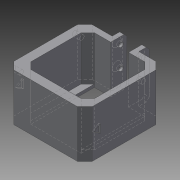
# Autodesk Inventor part: z-stepper holder
Saved by Autodesk Inventor 2015 (Build 190159000, 159)
## iProperties
Created: 2019-01-12
Part Number: z-stepper holder
Material: Generic
Document SubType Name: Modeling
Designer: Toby
Density: 1 g/cm^3
Appearance: Default
Author: Toby
Autodesk Inventor part; units mm, degrees
ref_plane "YZ Plane" through (0, 0, 0) normal (1, 0, 0) x (0, 1, 0)
ref_plane "XZ Plane" through (0, 0, 0) normal (0, 1, 0) x (-1, 0, 0)
ref_plane "XY Plane" through (0, 0, 0) normal (0, 0, 1) x (1, 0, 0)
sketch "Sketch1" plane through (0, 0, 0) normal (0, 0, 1) x (1, 0, 0)
  line L0 (-30.0725, 29.5446) -> (12.9275, 29.5446)
  line L1 (12.9275, 29.5446) -> (12.9275, -13.4554)
  line L2 (12.9275, -13.4554) -> (-30.0725, -13.4554)
  line L3 (-30.0725, -13.4554) -> (-30.0725, 29.5446)
  line L4 (-36.0725, 33.5446) -> (16.9275, 33.5446)
  line L5 (16.9275, 33.5446) -> (16.9275, -19.4554)
  line L6 (16.9275, -19.4554) -> (-36.0725, -19.4554)
  line L7 (-36.0725, -19.4554) -> (-36.0725, 33.5446)
  point P0 (0, 0)
  dimension "d0" = 43
  dimension "d1" = 43
  dimension "d2" = 6
  dimension "d3" = 4
  dimension "d4" = 6
  dimension "d5" = 4
  constraints: 16 end point, 4 parallel, 2 horizontal, 2 perpendicular
  measures "d0" distance of L2.end L0.start
  measures "d1" distance of L0.start L0.end
  measures "d2" distance between parallel lines of L7 L3
  measures "d3" distance between parallel lines of L5 L1
  measures "d4" distance between parallel lines of L6 L2
  measures "d5" distance between parallel lines of L4 L0
extrude "Extrusion1" add sketch "Sketch1" along normal blind 30
sketch "Sketch2" plane through (-36.0725, -19.4554, 0) normal (-1, 0, 0) x (0, 0, 1)
  line L0 (0, 0) -> (30, 0) projected
  point P0 (0, 19.4554)
  point P1 (25.9467, 5)
  point P2 (25.9467, 46)
  dimension "d8" = 5
  dimension "d9" = 41
  measures "d8" distance from line of L0 point (25.947, 5)
  measures "d9" distance of point (25.947, 5) point (25.947, 46)
hole "Hole1" at (-36.0725, -14.4554, 25.9467) at (-36.0725, 26.5446, 25.9467) direction (1, 0, 0) diameter 3 depth 5 tip angle 118
chamfer "Chamfer1" distance 4.5 angle 45 4 edges at (-30.0725, 29.5446, 15) (-30.0725, -13.4554, 15) (12.9275, -13.4554, 15) (12.9275, 29.5446, 15)
chamfer "Chamfer2" distance 5 angle 45 4 edges at (-36.0725, 33.5446, 15) (-36.0725, -19.4554, 15) (16.9275, -19.4554, 15) (16.9275, 33.5446, 15)
sketch "Sketch3" plane through (0, 0, 0) normal (0, 0, -1) x (-1, 0, 0)
  line L0 (-16.9275, 33.5446) -> (36.0725, 33.5446)
  line L1 (36.0725, 33.5446) -> (36.0725, -19.4554)
  line L2 (36.0725, -19.4554) -> (-16.9275, -19.4554)
  line L3 (-16.9275, -19.4554) -> (-16.9275, 33.5446)
  line L4 (31.0725, 33.5446) -> (-11.9275, 33.5446) projected
  line L5 (36.0725, -14.4554) -> (36.0725, 28.5446) projected
  line L6 (-11.9275, -19.4554) -> (31.0725, -19.4554) projected
  line L7 (-16.9275, 28.5446) -> (-16.9275, -14.4554) projected
  line L8 (-8.4275, 29.5446) -> (25.5725, 29.5446)
  line L9 (25.5725, 29.5446) -> (25.5725, -13.4554)
  line L10 (25.5725, -13.4554) -> (-8.4275, -13.4554)
  line L11 (-8.4275, -13.4554) -> (-8.4275, 29.5446)
  point P0 (0, 0)
  constraints: 16 end point, 4 collinear, 4 parallel, 2 horizontal, 2 perpendicular
extrude "Extrusion2" add sketch "Sketch3" along normal blind 2
chamfer "Chamfer3" distance 5 angle 45 4 edges at (16.9275, 33.5446, -1) (-36.0725, 33.5446, -1) (-36.0725, -19.4554, -1) (16.9275, -19.4554, -1)
sketch "Sketch4" plane through (-31.0725, 33.5446, 30) normal (0, 1, 0) x (1, 0, 0)
  line L0 (39.5, 32) -> (5.5, 32) projected
  line L1 (5.5, 0) -> (39.5, 0) projected
  line L2 (30, 32) -> (15, 32)
  line L3 (15, 32) -> (15, 0)
  line L4 (15, 0) -> (30, 0)
  line L5 (30, 0) -> (30, 32)
  point P0 (31.0725, 30)
  point P1 (22.5, 32)
  dimension "d28" = 15
  dimension "d29" = 7.5
  constraints: 8 end point, 2 parallel, 2 point on line, 1 horizontal, 1 midpoint, 1 perpendicular
  measures "d28" distance between parallel lines of L3 L5
  measures "d29" distance from line of point (22.5, 32) L5
extrude "Extrusion3" cut sketch "Sketch4" against normal blind 10
sketch "Sketch5" plane through (-36.0725, -14.4554, 30) normal (-1, 0, 0) x (0, 0, 1)
  line L0 (0, 5.5) -> (-30, 5.5) projected
  line L1 (-18.3238, 5.5) -> (-12.7551, 5.5)
  line L2 (-30, 1) -> (0, 1) projected
  line L3 (-15.5395, 1) -> (-18.3238, 5.5)
  line L4 (-12.7551, 5.5) -> (-15.5395, 1)
  line L5 (-18.3238, 5.5) -> (-12.7551, 5.5)
  point P0 (-30, 14.4554)
  constraints: 8 end point, 3 point on line, 1 collinear
extrude "Extrusion4" cut sketch "Sketch5" against normal blind 1
sketch "Sketch6" plane through (0, 0, 30) normal (0, 0, 1) x (1, 0, 0)
  line L0 (-25.5725, 29.5446) -> (-16.0725, 29.5446) projected
  line L1 (-17.5725, 29.5446) -> (-14.5725, 29.5446)
  line L2 (-14.5725, 29.5446) -> (-14.5725, 40.5446)
  line L3 (-14.5725, 40.5446) -> (-17.5725, 40.5446)
  line L4 (-17.5725, 40.5446) -> (-17.5725, 29.5446)
  line L5 (0.4275, 29.5446) -> (-2.5725, 29.5446)
  line L6 (-2.5725, 29.5446) -> (-2.5725, 40.5446)
  line L7 (-2.5725, 40.5446) -> (0.4275, 40.5446)
  line L8 (0.4275, 40.5446) -> (0.4275, 29.5446)
  line L9 (-16.0725, 29.5446) -> (-16.0725, 33.5446) projected
  line L10 (-1.0725, 33.5446) -> (-1.0725, 29.5446) projected
  line L11 (-16.0725, 33.5446) -> (-31.0725, 33.5446) projected
  point P0 (0, 0)
  dimension "d34" = 3
  dimension "d35" = 3
  dimension "d36" = 1.5
  dimension "d37" = 1.5
  dimension "d38" = 7
  constraints: 16 end point, 4 parallel, 3 point on line, 2 horizontal, 2 perpendicular
  measures "d34" distance between parallel lines of L2 L4
  measures "d35" distance between parallel lines of L8 L6
  measures "d36" distance between parallel lines of L9 L4
  measures "d37" distance between parallel lines of L10 L8
  measures "d38" distance between parallel lines of L11 L3
extrude "Extrusion5" add sketch "Sketch6" against normal blind 32
sketch "Sketch7" plane through (-17.5725, 33.5446, 30) normal (-1, 0, 0) x (0, 0, 1)
  line L0 (0, -4) -> (0, 7) projected
  line L1 (0, 7) -> (-32, 7) projected
  line L2 (-32, 0) -> (-32, 7) projected
  point P0 (-30, -33.5446)
  point P1 (-19, 3)
  point P2 (-5, 3)
  dimension "d41" = 5
  dimension "d42" = 4
  dimension "d43" = 4
  dimension "d44" = 13
  measures "d41" distance from line of L0 point (-5, 3)
  measures "d42" distance from line of L1 point (-5, 3)
  measures "d43" distance from line of L1 point (-19, 3)
  measures "d44" distance from line of L2 point (-19, 3)
hole "Hole2" at (-17.5725, 36.5446, 11) at (-17.5725, 36.5446, 25) direction (1, 0, 0) diameter 3 depth 8 tip angle 118 countersink diameter 6 countersink angle 90
chamfer "Chamfer4" distance 2 angle 45 4 edges at (-1.0725, 40.5446, -2) (-16.0725, 40.5446, -2) (-1.0725, 40.5446, 30) (-16.0725, 40.5446, 30)
sketch "Sketch8" plane through (0.4275, 33.5446, 30) normal (1, 0, 0) x (0, 0, -1)
  circle A0 centre (5, 3) radius 1.5 projected
  circle A1 centre (19, 3) radius 1.5 projected
  point P0 (30, -33.5446)
  constraints: 2 coincident
hole "Hole3" at (0.4275, 36.5446, 25) at (0.4275, 36.5446, 11) direction (-1, 0, 0) diameter 3 depth 8 tip angle 118
sketch "Sketch9" plane through (16.9275, -14.4554, 30) normal (1, 0, 0) x (0, 0, -1)
  line L0 (12.7551, 5.5) -> (18.3238, 5.5)
  line L1 (30, 5.5) -> (0, 5.5) projected
  line L2 (18.3238, 5.5) -> (15.5395, 1)
  line L3 (15.5395, 1) -> (18.3238, 5.5) projected
  line L4 (15.5395, 1) -> (12.7551, 5.5)
  line L5 (12.7551, 5.5) -> (15.5395, 1) projected
  point P0 (30, 14.4554)
  constraints: 6 end point, 3 collinear
extrude "Extrusion6" cut sketch "Sketch9" against normal blind 1
body "Solid1"
